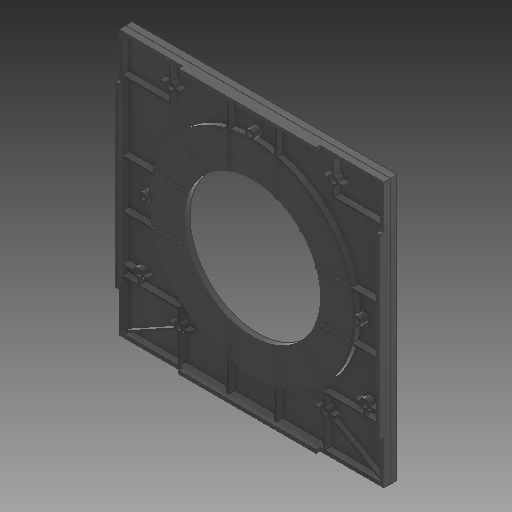
# Autodesk Inventor part: OSŁONA BLACHY CHWYTAJĄCEJ MONITOR
Saved by Autodesk Inventor 2017 SP1 (Build 210196100, 196)
## iProperties
Created: 2021-02-11
Part Number: OSŁONA BLACHY CHWYTAJĄCEJ MONITOR
Material: Tworzywo sztuczne, nieprzezroczyste czarne
Document SubType Name: Modeling
Designer: Napoleon
Mass: 36.9718 g
Surface Area: 337.315 cm^2
Volume: 38.8359 cm^3
Density: 0.952 g/cm^3
Appearance: Gładkie - czarne
Author: Napoleon
Autodesk Inventor part; units mm, degrees
ref_plane "YZ Plane" through (0, 0, 0) normal (1, 0, 0) x (0, 1, 0)
ref_plane "XZ Plane" through (0, 0, 0) normal (0, 1, 0) x (-1, 0, 0)
ref_plane "Płaszczyzna konstrukcyjna1" through (9.9155, -12.3592, 0) normal (0, 0, 1) x (1, 0, 0)
sketch "Szkic1" plane through (9.9155, -12.3592, 0) normal (0, 0, 1) x (1, 0, 0)
  circle A0 centre (-50.4806, 12.3592) radius 2.1 projected
  circle A1 centre (-50.4806, 49.7342) radius 1.6 projected
  circle A2 centre (-0.8306, 61.4048) radius 2.1 projected
  circle A3 centre (31.2194, 64.3342) radius 1.6 projected
  circle A4 centre (43.3694, 45.8092) radius 1.6 projected
  circle A5 centre (-50.4806, -25.0158) radius 1.6 projected
  arc A6 (-2.9306, -37.7158) -> (1.2694, -37.7158) centre (-0.8306, -37.7158) ccw projected
  arc A7 (1.2694, -35.6658) -> (-2.9306, -35.6658) centre (-0.8306, -35.6658) ccw projected
  arc A8 (-32.915, 57.825) -> (-33.815, 56.925) centre (-32.915, 56.925) ccw projected
  line L0 (-33.815, 44.975) -> (-33.815, 56.925) projected
  arc A9 (-34.915, 43.875) -> (-33.815, 44.975) centre (-34.915, 44.975) ccw projected
  line L1 (-58.1236, 43.875) -> (-34.915, 43.875) projected
  line L2 (-60.065, 41.9336) -> (-58.1236, 43.875) projected
  line L3 (-60.065, 34.0664) -> (-60.065, 41.9336) projected
  line L4 (-58.1236, 32.125) -> (-60.065, 34.0664) projected
  line L5 (-48.415, 32.125) -> (-58.1236, 32.125) projected
  line L6 (-48.415, -32.125) -> (-48.415, 32.125) projected
  line L7 (-58.1236, -32.125) -> (-48.415, -32.125) projected
  line L8 (-60.065, -34.0664) -> (-58.1236, -32.125) projected
  line L9 (-60.065, -41.9336) -> (-60.065, -34.0664) projected
  line L10 (-58.1236, -43.875) -> (-60.065, -41.9336) projected
  line L11 (-34.915, -43.875) -> (-58.1236, -43.875) projected
  arc A10 (-33.815, -44.975) -> (-34.915, -43.875) centre (-34.915, -44.975) ccw projected
  line L12 (-33.815, -56.925) -> (-33.815, -44.975) projected
  arc A11 (-33.815, -56.925) -> (-32.915, -57.825) centre (-32.915, -56.925) ccw projected
  line L13 (46.435, -57.825) -> (-32.915, -57.825) projected
  arc A12 (46.435, -57.825) -> (47.335, -56.925) centre (46.435, -56.925) ccw projected
  line L14 (47.335, -41) -> (47.335, -56.925) projected
  arc A13 (48.435, -39.9) -> (47.335, -41) centre (48.435, -41) ccw projected
  line L15 (62.485, -39.9) -> (48.435, -39.9) projected
  line L16 (62.485, -28.1) -> (62.485, -39.9) projected
  line L17 (61.385, -28.1) -> (62.485, -28.1) projected
  line L18 (61.385, 28.1) -> (61.385, -28.1) projected
  line L19 (62.485, 28.1) -> (61.385, 28.1) projected
  line L20 (62.485, 39.9) -> (62.485, 28.1) projected
  line L21 (48.435, 39.9) -> (62.485, 39.9) projected
  arc A14 (47.335, 41) -> (48.435, 39.9) centre (48.435, 41) ccw projected
  line L22 (47.335, 56.925) -> (47.335, 41) projected
  arc A15 (47.335, 56.925) -> (46.435, 57.825) centre (46.435, 56.925) ccw projected
  line L23 (-32.915, 57.825) -> (46.435, 57.825) projected
  circle A16 centre (-40.565, 0) radius 2.1 projected
  circle A17 centre (-40.565, -37.375) radius 1.6 projected
  circle A18 centre (-40.565, 37.375) radius 1.6 projected
  circle A19 centre (41.135, 51.975) radius 1.6 projected
  circle A20 centre (41.135, -51.975) radius 1.6 projected
  circle A21 centre (53.285, 33.45) radius 1.6 projected
  circle A22 centre (53.285, -33.45) radius 1.6 projected
  arc A23 (-2.9306, -37.7158) -> (1.2694, -37.7158) centre (9.085, -50.075) ccw projected
  line L24 (6.985, -37.7158) -> (6.985, -35.6658) projected
  arc A24 (1.2694, -35.6658) -> (-2.9306, -35.6658) centre (9.085, -48.025) ccw projected
  line L25 (11.185, -35.6658) -> (11.185, -37.7158) projected
  circle A25 centre (9.085, 46.925) radius 2.1 projected
  point P0 (-9.9155, 12.3592)
  constraints: 2 other
ref_plane "Płaszczyzna konstrukcyjna2" through (9.9155, -12.3592, 0.35) normal (0, 0, 1) x (1, 0, 0)
sketch "Szkic2" plane through (9.9155, -12.3592, 0.35) normal (0, 0, 1) x (1, 0, 0)
  circle A0 centre (9.085, 0) radius 31.25
  circle A1 centre (9.085, 0) radius 45.45
  point P0 (-9.9155, 12.3592)
  dimension "d1" = 62.5
  dimension "d2" = 90.9
  constraints: 2 centre point, 2 coincident
  measures "d1" diameter of A0
  measures "d2" diameter of A1
extrude "Wyciągnięcie proste1" add sketch "Szkic2" along normal blind 1.4
sketch "Szkic3" plane through (19.0005, -12.3592, 1.75) normal (0, 0, 1) x (1, 0, 0)
  circle A0 centre (0, 0) radius 45.45
  line L0 (60.8, -60.8) -> (-60.8, -60.8)
  line L1 (-60.8, -60.8) -> (-60.8, 60.8)
  line L2 (-60.8, 60.8) -> (60.8, 60.8)
  line L3 (60.8, 60.8) -> (60.8, -60.8)
  line L4 (60.8, -60.8) -> (-60.8, 60.8) construction
  line L5 (-60.8, -60.8) -> (60.8, 60.8) construction
  point P0 (-19.0005, 12.3592)
  dimension "d5" = 121.6
  dimension "d6" = 121.6
  constraints: 12 end point, 2 midpoint, 2 parallel, 1 centre point, 1 horizontal, 1 perpendicular
  measures "d5" distance of L1.end L2.end
  measures "d6" distance of L0.end L1.end
extrude "Wyciągnięcie proste2" add sketch "Szkic3" along normal blind 3
sketch "Szkic4" plane through (19.0005, -12.3592, 1.75) normal (0, 0, -1) x (-1, 0, 0)
  circle A0 centre (0, 0) radius 45.45 projected
  line L0 (-60.75, 60.75) -> (60.75, 60.75)
  line L1 (60.75, 60.75) -> (60.75, -60.75)
  line L2 (60.75, -60.75) -> (-60.75, -60.75)
  line L3 (-60.75, -60.75) -> (-60.75, 60.75)
  line L4 (-59.25, -59.25) -> (59.25, -59.25)
  line L5 (59.25, -59.25) -> (59.25, 59.25)
  line L6 (59.25, 59.25) -> (-59.25, 59.25)
  line L7 (-59.25, 59.25) -> (-59.25, -59.25)
  line L8 (-59.25, -59.25) -> (59.25, 59.25) construction
  line L9 (59.25, -59.25) -> (-59.25, 59.25) construction
  point P0 (-60.8, -60.8)
  point P1 (60.8, 60.8)
  dimension "d11" = 121.5
  dimension "d12" = 121.5
  dimension "d13" = 118.5
  dimension "d14" = 118.5
  constraints: 20 end point, 4 parallel, 2 horizontal, 2 midpoint, 2 perpendicular
  measures "d11" distance of L1.end L2.end
  measures "d12" distance of L0.end L1.end
  measures "d13" distance of L6.end L5.end
  measures "d14" distance of L5.end L4.end
extrude "Wyciągnięcie proste3" add sketch "Szkic4" along normal blind 3 contours L0 L1 L2 L3
sketch "Szkic5" plane through (19.0005, -12.3592, -1.25) normal (0, 0, -1) x (-1, 0, 0)
  line L0 (59.25, -31.5) -> (59.25, 31.5)
  line L1 (60.75, -31.5) -> (60.75, 31.5)
  line L2 (60.75, 31.5) -> (59.25, 31.5)
  line L3 (60.75, -31.5) -> (59.25, -31.5)
  line L4 (-59.25, -31.5) -> (-59.25, 31.5)
  line L5 (-60.75, -31.5) -> (-60.75, 31.5)
  line L6 (-60.75, 31.5) -> (-59.25, 31.5)
  line L7 (-60.75, -31.5) -> (-59.25, -31.5)
  line L8 (-40.75, 60.75) -> (40.75, 60.75)
  line L9 (40.75, 60.75) -> (40.75, 59.25)
  line L10 (-40.75, 60.75) -> (-40.75, 59.25)
  line L11 (-40.75, 59.25) -> (40.75, 59.25)
  line L12 (-40.75, -60.75) -> (40.75, -60.75)
  line L13 (40.75, -60.75) -> (40.75, -59.25)
  line L14 (-40.75, -60.75) -> (-40.75, -59.25)
  line L15 (-40.75, -59.25) -> (40.75, -59.25)
  constraints: 32 end point, 2 perpendicular
extrude "Wyciągnięcie proste4" add sketch "Szkic5" along normal blind 1.85
sketch "Szkic6" plane through (19.0005, -12.3592, 1.75) normal (0, 0, -1) x (-1, 0, 0)
  circle A0 centre (49.65, 37.3931) radius 1.5
  circle A1 centre (49.65, -37.375) radius 1.5
  circle A2 centre (-44.2, 33.45) radius 1.5
  circle A3 centre (-32.05, 51.975) radius 1.5
  line L0 (59.25, 37.7931) -> (51.8133, 37.7931)
  line L1 (51.8133, 36.9931) -> (59.25, 36.9931)
  line L2 (59.25, 37.7931) -> (59.25, 36.9931)
  line L3 (59.25, -37.7931) -> (51.8099, -37.7931)
  line L4 (51.8133, -36.9931) -> (59.25, -36.9931)
  line L5 (59.25, -37.7931) -> (59.25, -36.9931)
  line L6 (43.45, 59.25) -> (43.45, 37.7931)
  line L7 (43.45, 37.7931) -> (47.4867, 37.7931)
  line L8 (47.4867, 36.9931) -> (42.65, 36.9931)
  line L9 (42.65, 59.25) -> (42.65, 36.9931)
  line L10 (43.45, 59.25) -> (42.65, 59.25)
  line L11 (43.45, -59.25) -> (43.45, -37.7931)
  line L12 (43.45, -37.7931) -> (47.4901, -37.7931)
  line L13 (47.4867, -36.9931) -> (42.65, -36.9931)
  line L14 (42.65, -59.25) -> (42.65, -36.9931)
  line L15 (43.45, -59.25) -> (42.65, -59.25)
  line L16 (59.25, 11.3931) -> (45.8559, 11.3931)
  line L17 (59.25, 11.3931) -> (59.25, 10.5931)
  line L18 (59.25, 10.5931) -> (46.0579, 10.5467)
  line L19 (59.25, -11.3931) -> (45.8559, -11.3931)
  line L20 (59.25, -11.3931) -> (59.25, -10.5931)
  line L21 (59.25, -10.5931) -> (46.0579, -10.5467)
  line L22 (-59.25, 33.6544) -> (-59.25, 33.1956)
  line L23 (-46.3861, 33.6972) -> (-59.25, 33.6544)
  line L24 (-46.3852, 33.1956) -> (-59.25, 33.1956)
  line L25 (-42.0148, 33.1956) -> (-36.3, 33.1956)
  line L26 (-37.1, 33.7436) -> (-42.0197, 33.7436)
  line L27 (49.25, 42.1431) -> (50.05, 42.1431)
  line L28 (50.05, 32.6431) -> (49.25, 32.6431)
  line L29 (50.05, 42.1431) -> (50.05, 39.5564)
  line L30 (49.25, 39.5564) -> (49.25, 42.1431)
  line L31 (49.25, 32.6431) -> (49.25, 35.2298)
  line L32 (50.05, 35.2298) -> (50.05, 32.6431)
  arc A4 (51.8133, 37.7931) -> (50.05, 39.5564) centre (49.65, 37.3931) ccw
  arc A5 (49.25, 39.5564) -> (47.4867, 37.7931) centre (49.65, 37.3931) ccw
  arc A6 (47.4867, 36.9931) -> (49.25, 35.2298) centre (49.65, 37.3931) ccw
  arc A7 (50.05, 35.2298) -> (51.8133, 36.9931) centre (49.65, 37.3931) ccw
  line L33 (49.25, -42.1431) -> (50.0468, -42.1431)
  line L34 (50.05, -32.6431) -> (49.25, -32.6431)
  line L35 (50.0468, -42.1431) -> (50.0468, -39.5389)
  line L36 (49.25, -39.5383) -> (49.25, -42.1431)
  line L37 (49.25, -32.6431) -> (49.25, -35.2298)
  line L38 (50.05, -35.2298) -> (50.05, -32.6431)
  arc A8 (47.4901, -37.7931) -> (49.25, -39.5383) centre (49.65, -37.375) ccw
  arc A9 (50.0468, -39.5389) -> (51.8099, -37.7931) centre (49.65, -37.375) ccw
  arc A10 (51.8166, -36.9931) -> (50.05, -35.2117) centre (49.65, -37.375) ccw
  arc A11 (49.25, -35.2117) -> (47.4834, -36.9931) centre (49.65, -37.375) ccw
  line L39 (-37.1, 59.25) -> (-37.1, 33.7436)
  line L40 (-36.3, 59.25) -> (-37.1, 59.25)
  line L41 (-34.2133, 51.575) -> (-36.3, 51.575)
  line L42 (-34.2133, 52.375) -> (-36.3, 52.375)
  line L43 (-36.3, 59.25) -> (-36.3, 52.375)
  line L44 (-36.3, 51.575) -> (-36.3, 33.1956)
  line L45 (-31.65, 59.25) -> (-32.45, 59.25)
  line L46 (-32.45, 59.25) -> (-32.45, 54.1383)
  line L47 (-31.65, 54.1383) -> (-31.65, 59.25)
  arc A12 (-32.45, 54.1383) -> (-34.2133, 52.375) centre (-32.05, 51.975) ccw
  line L48 (-31.65, 47.6251) -> (-32.45, 47.6251)
  line L49 (-31.65, 49.8117) -> (-31.65, 47.6251)
  line L50 (-32.45, 47.6251) -> (-32.45, 49.8117)
  arc A13 (-34.2133, 51.575) -> (-32.45, 49.8117) centre (-32.05, 51.975) ccw
  arc A14 (-31.65, 49.8117) -> (-31.65, 54.1383) centre (-32.05, 51.975) ccw
  line L51 (-44.6, 38.2) -> (-43.8, 38.2)
  line L52 (-43.8, 28.7) -> (-44.6, 28.7)
  line L53 (-43.8, 38.2) -> (-43.8, 35.6133)
  line L54 (-44.6, 35.6133) -> (-44.6, 38.2)
  line L55 (-44.6, 28.7) -> (-44.6, 31.2867)
  line L56 (-43.8, 31.2867) -> (-43.8, 28.7)
  arc A15 (-42.0197, 33.7436) -> (-43.8, 35.6133) centre (-44.2, 33.45) ccw
  arc A16 (-44.6, 35.6133) -> (-46.3861, 33.6972) centre (-44.2, 33.45) ccw
  arc A17 (-46.3852, 33.1956) -> (-44.6, 31.2867) centre (-44.2, 33.45) ccw
  arc A18 (-43.8, 31.2867) -> (-42.0148, 33.1956) centre (-44.2, 33.45) ccw
  circle A19 centre (-44.2, -33.45) radius 1.5
  circle A20 centre (-32.05, -51.975) radius 1.5
  line L57 (-46.3861, -33.6972) -> (-59.25, -33.6544)
  line L58 (-46.3852, -33.1956) -> (-59.25, -33.1956)
  line L59 (-42.0148, -33.1956) -> (-36.3, -33.1956)
  line L60 (-37.1, -33.7436) -> (-42.0197, -33.7436)
  line L61 (-37.1, -59.25) -> (-37.1, -33.7436)
  line L62 (-36.3, -59.25) -> (-37.1, -59.25)
  line L63 (-34.2133, -51.575) -> (-36.3, -51.575)
  line L64 (-34.2133, -52.375) -> (-36.3, -52.375)
  line L65 (-36.3, -59.25) -> (-36.3, -52.375)
  line L66 (-36.3, -51.575) -> (-36.3, -33.1956)
  line L67 (-31.65, -59.25) -> (-32.45, -59.25)
  line L68 (-32.45, -59.25) -> (-32.45, -54.1383)
  line L69 (-31.65, -54.1383) -> (-31.65, -59.25)
  arc A21 (-34.2133, -52.375) -> (-32.45, -54.1383) centre (-32.05, -51.975) ccw
  line L70 (-31.65, -47.6251) -> (-32.45, -47.6251)
  line L71 (-31.65, -49.8117) -> (-31.65, -47.6251)
  line L72 (-32.45, -47.6251) -> (-32.45, -49.8117)
  arc A22 (-32.45, -49.8117) -> (-34.2133, -51.575) centre (-32.05, -51.975) ccw
  arc A23 (-31.65, -54.1383) -> (-31.65, -49.8117) centre (-32.05, -51.975) ccw
  line L73 (-44.6, -28.7) -> (-44.6, -31.2867)
  line L74 (-43.8, -28.7) -> (-44.6, -28.7)
  line L75 (-43.8, -31.2867) -> (-43.8, -28.7)
  line L76 (-44.6, -38.2) -> (-43.8, -38.2)
  line L77 (-43.8, -38.2) -> (-43.8, -35.6133)
  line L78 (-44.6, -35.6133) -> (-44.6, -38.2)
  arc A24 (-43.8, -35.6133) -> (-42.0197, -33.7436) centre (-44.2, -33.45) ccw
  arc A25 (-46.3861, -33.6972) -> (-44.6, -35.6133) centre (-44.2, -33.45) ccw
  arc A26 (-44.6, -31.2867) -> (-46.3852, -33.1956) centre (-44.2, -33.45) ccw
  arc A27 (-42.0148, -33.1956) -> (-43.8, -31.2867) centre (-44.2, -33.45) ccw
  line L79 (-59.25, -33.1956) -> (-59.25, -33.6544)
  arc A28 (46.0579, 10.5467) -> (45.8559, 11.3931) centre (0, 0) ccw
  arc A29 (45.8559, -11.3931) -> (46.0579, -10.5467) centre (0, 0) ccw
  line L80 (-11.3931, 59.25) -> (-10.5931, 59.25)
  line L81 (-10.5931, 59.25) -> (-10.5467, 46.0579)
  line L82 (10.5931, 59.25) -> (10.5467, 46.0579)
  line L83 (11.3931, 59.25) -> (11.3931, 45.8559)
  line L84 (11.3931, 59.25) -> (10.5931, 59.25)
  arc A30 (11.3931, 45.8559) -> (10.5467, 46.0579) centre (0, 0) ccw
  arc A31 (-10.5467, 46.0579) -> (-11.3931, 45.8559) centre (0, 0) ccw
  line L85 (-11.3931, 59.25) -> (-11.3931, 45.8559)
  line L86 (-59.25, -11.3931) -> (-59.25, -10.5931)
  line L87 (-59.25, -10.5931) -> (-46.0579, -10.5467)
  line L88 (-59.25, 10.5931) -> (-46.0579, 10.5467)
  line L89 (-59.25, 11.3931) -> (-45.8559, 11.3931)
  line L90 (-59.25, 11.3931) -> (-59.25, 10.5931)
  arc A32 (-45.8559, 11.3931) -> (-46.0579, 10.5467) centre (0, 0) ccw
  arc A33 (-46.0579, -10.5467) -> (-45.8559, -11.3931) centre (0, 0) ccw
  line L91 (-59.25, -11.3931) -> (-45.8559, -11.3931)
  line L92 (11.3931, -59.25) -> (10.5931, -59.25)
  line L93 (10.5931, -59.25) -> (10.5467, -46.0579)
  line L94 (-10.5931, -59.25) -> (-10.5467, -46.0579)
  line L95 (-11.3931, -59.25) -> (-11.3931, -45.8559)
  line L96 (-11.3931, -59.25) -> (-10.5931, -59.25)
  arc A34 (-11.3931, -45.8559) -> (-10.5467, -46.0579) centre (0, 0) ccw
  arc A35 (10.5467, -46.0579) -> (11.3931, -45.8559) centre (0, 0) ccw
  line L97 (11.3931, -59.25) -> (11.3931, -45.8559)
  point P0 (55.5126, 37.375)
  point P1 (55.5126, -37.375)
  point P2 (-32.4501, -49.8117)
  dimension "d35" = 0.8
  dimension "d39" = 0.8
  dimension "d45" = 0.8
  dimension "d55" = 0.8
  dimension "d59" = 0.8
  dimension "d62" = 0.8
  dimension "d71" = 360
  dimension "d109" = 3
  dimension "d110" = 3
  dimension "d111" = 3
  dimension "d112" = 3
  dimension "d113" = 3
  dimension "d114" = 3
  constraints: 197 end point, 60 point on circle, 36 centre point, 11 parallel, 11 perpendicular, 6 coincident, 4 point on line, 3 horizontal, 1 vertical, 69 other
  measures "d35" distance of L1.start L0.end
  measures "d39" distance of L16.start L17.end
  measures "d45" distance of L27.start L27.end
  measures "d55" distance of L39.start L40.start
  measures "d59" distance of L45.start L45.end
  measures "d62" distance of L51.start L51.end
  measures "d109" diameter of A20
  measures "d110" diameter of A2
  measures "d111" diameter of A19
  measures "d112" diameter of A3
  measures "d113" diameter of A0
  measures "d114" diameter of A1
extrude "Wyciągnięcie proste5" add sketch "Szkic6" along normal blind 3
sketch "Szkic7" plane through (9.9155, -12.3592, 0.35) normal (0, 0, -1) x (-1, 0, 0)
  circle A0 centre (-9.085, 0) radius 31.25
  circle A1 centre (-9.085, 0) radius 47.25
  point P0 (9.9155, 12.3592)
  dimension "d46" = 94.5
  constraints: 2 centre point, 1 coincident
  measures "d46" diameter of A1
extrude "Wyciągnięcie proste6" add sketch "Szkic7" against normal blind 1.4 and the other way blind 1.1
sketch "Szkic8" plane through (9.9155, -12.3592, -0.75) normal (0, 0, -1) x (-1, 0, 0)
  arc A0 (36.9924, 10.5515) -> (36.7916, 11.3931) centre (-9.0655, 0.0048) ccw
  line L0 (36.7916, 11.3931) -> (20.0142, 11.3931)
  line L1 (36.9924, 10.5515) -> (20.351, 10.5515)
  arc A1 (20.351, 10.5515) -> (20.0142, 11.3931) centre (-8.8266, -0.6391) ccw
  arc A2 (36.7916, -11.3931) -> (36.9924, -10.5515) centre (-9.0655, -0.0048) ccw
  line L2 (36.7916, -11.3931) -> (20.0142, -11.3931)
  line L3 (36.9924, -10.5515) -> (20.351, -10.5515)
  arc A3 (20.0142, -11.3931) -> (20.351, -10.5515) centre (-8.8266, 0.6391) ccw
  arc A4 (-19.6365, 46.0774) -> (-20.4781, 45.8766) centre (-9.0898, 0.0195) ccw
  line L4 (-20.4781, 45.8766) -> (-20.4781, 29.0991)
  line L5 (-19.6365, 46.0774) -> (-19.6365, 29.436)
  arc A5 (-19.6365, 29.436) -> (-20.4781, 29.0991) centre (-8.4459, 0.2584) ccw
  arc A6 (2.3081, 45.8766) -> (1.4666, 46.0774) centre (-9.0801, 0.0195) ccw
  line L6 (2.3081, 45.8766) -> (2.3081, 29.0991)
  line L7 (1.4666, 46.0774) -> (1.4666, 29.436)
  arc A7 (2.3081, 29.0991) -> (1.4666, 29.436) centre (-9.724, 0.2584) ccw
  arc A8 (-55.1624, -10.5515) -> (-54.9615, -11.3931) centre (-9.1045, -0.0048) ccw
  line L8 (-54.9615, -11.3931) -> (-38.1841, -11.3931)
  line L9 (-55.1624, -10.5515) -> (-38.521, -10.5515)
  arc A9 (-38.521, -10.5515) -> (-38.1841, -11.3931) centre (-9.3433, 0.6391) ccw
  arc A10 (-54.9615, 11.3931) -> (-55.1624, 10.5515) centre (-9.1045, 0.0048) ccw
  line L10 (-54.9615, 11.3931) -> (-38.1841, 11.3931)
  line L11 (-55.1624, 10.5515) -> (-38.521, 10.5515)
  arc A11 (-38.1841, 11.3931) -> (-38.521, 10.5515) centre (-9.3433, -0.6391) ccw
  arc A12 (1.4666, -46.0774) -> (2.3081, -45.8766) centre (-9.0801, -0.0195) ccw
  line L12 (2.3081, -45.8766) -> (2.3081, -29.0991)
  line L13 (1.4666, -46.0774) -> (1.4666, -29.436)
  arc A13 (1.4666, -29.436) -> (2.3081, -29.0991) centre (-9.724, -0.2584) ccw
  arc A14 (-20.4781, -45.8766) -> (-19.6365, -46.0774) centre (-9.0898, -0.0195) ccw
  line L14 (-20.4781, -45.8766) -> (-20.4781, -29.0991)
  line L15 (-19.6365, -46.0774) -> (-19.6365, -29.436)
  arc A15 (-20.4781, -29.0991) -> (-19.6365, -29.436) centre (-8.4459, -0.2584) ccw
  line L16 (24.0418, 33.6924) -> (12.7275, 22.3781)
  line L17 (13.2932, 21.8124) -> (24.6075, 33.1268)
  arc A16 (13.2932, 21.8124) -> (12.7275, 22.3781) centre (-9.085, 0) ccw
  arc A17 (2.3081, 29.0991) -> (20.0142, 11.3931) centre (-9.085, 0) ccw
  arc A18 (24.6075, 33.1268) -> (24.0418, 33.6924) centre (-9.085, 0) ccw
  arc A19 (36.7709, -11.3931) -> (36.9729, -10.5467) centre (-9.085, 0) ccw projected
  arc A20 (-30.8974, 22.3781) -> (-31.4631, 21.8124) centre (-9.085, 0) ccw
  line L18 (-30.8974, 22.3781) -> (-42.2117, 33.6924)
  line L19 (-42.7774, 33.1268) -> (-31.4631, 21.8124)
  arc A21 (-42.2117, 33.6924) -> (-42.7774, 33.1268) centre (-9.085, 0) ccw
  arc A22 (-31.4631, -21.8124) -> (-30.8974, -22.3781) centre (-9.085, 0) ccw
  line L20 (-31.4631, -21.8124) -> (-42.7774, -33.1268)
  line L21 (-42.2117, -33.6924) -> (-30.8974, -22.3781)
  arc A23 (-42.7774, -33.1268) -> (-42.2117, -33.6924) centre (-9.085, 0) ccw
  arc A24 (12.7275, -22.3781) -> (13.2932, -21.8124) centre (-9.085, 0) ccw
  line L22 (12.7275, -22.3781) -> (24.0418, -33.6924)
  line L23 (24.6075, -33.1268) -> (13.2932, -21.8124)
  arc A25 (24.0418, -33.6924) -> (24.6075, -33.1268) centre (-9.085, 0) ccw
  point P0 (-9.085, 0)
  dimension "d79" = 360
  dimension "d92" = 360
  constraints: 50 point on circle, 48 end point, 25 centre point, 1 coincident, 1 horizontal, 122 other
extrude "Wyciągnięcie proste7" add sketch "Szkic8" along normal up to surface (0.5 mm away)
sketch "Szkic9" plane through (19.0005, -12.3592, 1.75) normal (0, 0, -1) x (-1, 0, 0)
  line L0 (-59.25, -58.434) -> (-46.071, -34.6072)
  line L1 (-45.503, -35.2226) -> (-58.7929, -59.25)
  arc A0 (-46.071, -34.6072) -> (-45.503, -35.2226) centre (-44.2, -33.45) ccw
  line L2 (-58.7929, -59.25) -> (-59.25, -59.25)
  line L3 (-59.25, -59.25) -> (-59.25, -58.434)
  line L4 (-59.25, 58.434) -> (-46.071, 34.6072)
  line L5 (-45.503, 35.2226) -> (-58.7929, 59.25)
  arc A1 (-45.503, 35.2226) -> (-46.071, 34.6072) centre (-44.2, 33.45) ccw
  line L6 (-58.7929, 59.25) -> (-59.25, 59.25)
  line L7 (-59.25, 59.25) -> (-59.25, 58.434)
  point P0 (-46.3861, -33.6972)
  point P1 (19.0005, 12.3592)
  point P2 (-52.5297, -47.1)
  point P3 (-46.3861, 33.6972)
  point P4 (-52.5297, 47.1)
  constraints: 16 end point, 4 point on circle, 2 centre point, 1 horizontal, 1 parallel, 1 perpendicular
extrude "Wyciągnięcie proste8" add sketch "Szkic9" along normal blind 2.2
sketch "Szkic10" plane through (19.0005, -12.3592, 1.75) normal (0, 0, -1) x (-1, 0, 0)
  circle A0 centre (49.65, 0) radius 2
  circle A1 centre (0, 49.0457) radius 2
  circle A2 centre (49.65, 0) radius 1.1
  circle A3 centre (0, 49.0457) radius 1.1
  circle A4 centre (0, -49.05) radius 1.1
  circle A5 centre (0, -49.05) radius 2
  point P0 (19.0005, 12.3592)
  dimension "d97" = 2.2
  dimension "d99" = 2.2
  dimension "d127" = 2.2
  dimension "d128" = 4
  dimension "d129" = 4
  dimension "d130" = 4
  constraints: 6 centre point, 3 coincident
  measures "d97" diameter of A2
  measures "d99" diameter of A4
  measures "d127" diameter of A3
  measures "d128" diameter of A1
  measures "d129" diameter of A0
  measures "d130" diameter of A5
extrude "Wyciągnięcie proste9" add sketch "Szkic10" along normal blind 3.75
thread "Gwint4" size "M3x0.5" class "6H" standard "ANSI Metric M Profile" full length
thread "Gwint5" size "M3x0.5" class "6H" standard "ANSI Metric M Profile" full length
thread "Gwint6" size "M3x0.5" class "6H" standard "ANSI Metric M Profile" full length
thread "Gwint7" size "M3x0.5" class "6H" standard "ANSI Metric M Profile" full length
thread "Gwint8" size "M3x0.5" class "6H" standard "ANSI Metric M Profile" full length
thread "Gwint9" size "M3x0.5" class "6H" standard "ANSI Metric M Profile" full length
